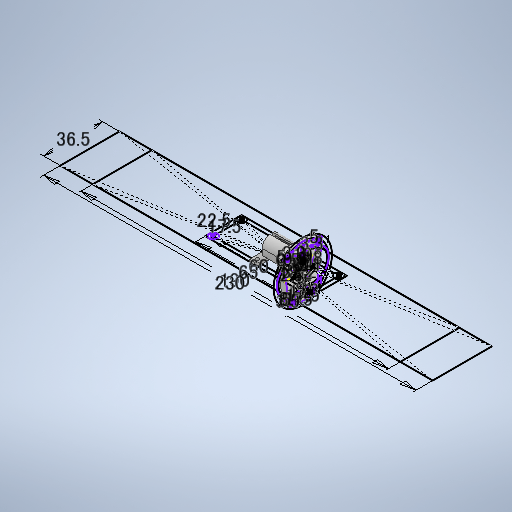
# Autodesk Inventor part: ikafly1
Saved by Autodesk Inventor 2025 (Build 290162000, 162)
## iProperties
Created: 2024-05-10
Part Number: ikafly1
Material: 一般
Document SubType Name: Modeling
Designer: Saigusa
Density: 1 g/cm^3
Appearance: 既定
Author: Saigusa
Autodesk Inventor part; units mm, degrees
ref_plane "YZ Plane" through (0, 0, 0) normal (1, 0, 0) x (0, 1, 0)
ref_plane "XZ Plane" through (0, 0, 0) normal (0, 1, 0) x (-1, 0, 0)
ref_plane "XY Plane" through (0, 0, 0) normal (0, 0, 1) x (1, 0, 0)
sketch "スケッチ2" plane through (0, 0, 0) normal (0, 1, 0) x (-1, 0, 0)
  line L0 (-32.5, -11.25) -> (32.5, -11.25)
  line L1 (32.5, -11.25) -> (32.5, 11.25)
  line L2 (32.5, 11.25) -> (-32.5, 11.25)
  line L3 (-32.5, 11.25) -> (-32.5, -11.25)
  line L4 (-32.5, -11.25) -> (32.5, 11.25) construction
  line L5 (32.5, -11.25) -> (-32.5, 11.25) construction
  line L6 (-30, -8.75) -> (30, -8.75)
  line L7 (30, -8.75) -> (30, 8.75)
  line L8 (30, 8.75) -> (-30, 8.75)
  line L9 (-30, 8.75) -> (-30, -8.75)
  line L10 (-30, -8.75) -> (30, 8.75) construction
  line L11 (30, -8.75) -> (-30, 8.75) construction
  circle A0 centre (30, 8.75) radius 2.5
  circle A1 centre (30, -8.75) radius 2.5
  circle A2 centre (-30, 8.75) radius 2.5
  circle A3 centre (-30, -8.75) radius 2.5
  line L12 (-115, -18.25) -> (115, -18.25)
  line L13 (115, -18.25) -> (115, 18.25)
  line L14 (115, 18.25) -> (-115, 18.25)
  line L15 (-115, 18.25) -> (-115, -18.25)
  line L16 (-115, -18.25) -> (115, 18.25) construction
  line L17 (115, -18.25) -> (-115, 18.25) construction
  line L18 (-95, -18.25) -> (95, -18.25)
  line L19 (95, -18.25) -> (95, 18.25)
  line L20 (95, 18.25) -> (-95, 18.25)
  line L21 (-95, 18.25) -> (-95, -18.25)
  line L22 (-95, -18.25) -> (95, 18.25) construction
  line L23 (95, -18.25) -> (-95, 18.25) construction
  point P0 (0, 0)
  dimension "d10" = 65
  dimension "d11" = 22.5
  dimension "d12" = 60
  dimension "d13" = 17.5
  dimension "d14" = 230
  dimension "d15" = 36.5
  dimension "d16" = 190
  constraints: 48 end point, 8 midpoint, 8 parallel, 4 centre point, 4 horizontal, 4 perpendicular, 4 tangent, 3 coincident, 1 point on line
  measures "d10" distance of L2.end L1.end
  measures "d11" distance of L1.end L0.end
  measures "d12" distance of L8.end L7.end
  measures "d13" distance of L7.end L6.end
  measures "d14" distance of L14.end L13.end
  measures "d15" distance of L13.end L12.end
  measures "d16" distance of L20.end L19.end
sketch "スケッチ4" plane through (0, 0, 0) normal (1, 0, 0) x (0, 1, 0)
  point P0 (0, 0)
sketch "スケッチ5" plane through (0, 0, 0) normal (1, 0, 0) x (0, 1, 0)
  circle A0 centre (0, 0) radius 18.25
  line L0 (0, 0) -> (0, 6)
  line L1 (0, 6) -> (0, -6)
  circle A1 centre (0, 6) radius 3
  circle A2 centre (0, -6) radius 9
  circle A3 centre (0, 6) radius 9
  circle A4 centre (0, -6) radius 3
  line L2 (0, 6) -> (5.2915, 0)
  circle A5 centre (5.2915, 0) radius 5
  circle A6 centre (5.2915, 0) radius 4.5
  circle A7 centre (5.2915, 0) radius 5.5
  line L3 (0, 0) -> (0, 11.25)
  line L4 (0, 11.25) -> (0, -11.25)
  line L5 (5.2915, 5.5) -> (5.2915, -5.5)
  line L6 (0, 11.25) -> (-1.2, 11.25)
  line L7 (-1.2, 11.25) -> (-1.2, -11.25)
  line L8 (-1.2, -11.25) -> (0, -11.25)
  line L9 (-1.2, 11.25) -> (-9.2, 11.25)
  line L10 (-1.2, -11.25) -> (-9.2, -11.25)
  line L11 (-9.2, -11.25) -> (-9.2, 11.25)
  line L12 (-9.2, 11.25) -> (-10.4, 11.25)
  line L13 (-10.4, 11.25) -> (-10.4, -11.25)
  line L14 (-10.4, -11.25) -> (-9.2, -11.25)
  circle A8 centre (0, 0) radius 16
  line L15 (0, 11.25) -> (1.5, 11.25)
  line L16 (1.5, 11.25) -> (1.5, -11.25)
  line L17 (1.5, -11.25) -> (0, -11.25)
  line L18 (5.2915, 5.5) -> (1.5, 5.5)
  line L19 (5.2915, -5.5) -> (1.5, -5.5)
  circle A9 centre (5.2915, 0) radius 6.6802
  point P0 (0, 1.5)
  point P1 (0, -1.5)
  point P2 (1.5, -3.9843)
  point P3 (1.5, 3.9843)
  dimension "d28" = 36.5
  dimension "d29" = 6
  dimension "d30" = 12
  dimension "d31" = 6
  dimension "d32" = 18
  dimension "d33" = 8
  dimension "d34" = 9
  dimension "d35" = 11
  dimension "d36" = 11.25
  dimension "d37" = 22.5
  dimension "d39" = 1.2
  dimension "d40" = 8
  dimension "d41" = 1.2
  dimension "d42" = 32
  dimension "d43" = 1.5
  constraints: 40 end point, 10 coincident, 9 centre point, 8 perpendicular, 7 point on line, 3 parallel, 3 point on circle, 3 tangent, 1 horizontal, 1 vertical, 3 other
  measures "d28" diameter of A0
  measures "d29" distance of L0.start L0.end
  measures "d30" distance of L0.end L1.end
  measures "d31" diameter of A1
  measures "d32" diameter of A3
  measures "d33" distance of L2.start L2.end
  measures "d34" diameter of A6
  measures "d35" diameter of A7
  measures "d36" distance of L0.start L3.end
  measures "d37" distance of L3.end L4.end
  measures "d39" distance of L3.end L6.end
  measures "d40" distance of L6.end L9.end
  measures "d41" distance of L9.end L12.end
  measures "d42" diameter of A8
  measures "d43" distance of L3.end L15.end
extrude "押し出し1" add sketch "スケッチ5" against normal blind 5 contours L0 A7 A2 A5 A3 L1 | L0 A2 A7 | A7 A3 L1 | L0 A9 L2 L16 A7 A1 | A1 A7 A2 | A7 A1 L16 A5 A2 | A4 A7 L16 A9 L1 | A3 A7 A4 | A3 A5 L16 A4 A7 | L0 L2 A9 | A7 L16 A1 | A5 L16 A2 | A2 L16 A6 A3 A5 | A9 L16 A4 L4 L1 | A4 L16 A7 | A3 L16 A5 | L3 A1 L16 A9 L2 | A9 L16 L2 | L3 L15 L16 A1 | L16 A6 | A4 L16 L17 L4 picked at (1.4091, -3.6973)
extrude "押し出し2" add sketch "スケッチ5" against normal blind 3 contours L0 A7 A2 A5 A3 L1 | A7 A1 L16 A5 A2 | A3 A5 L16 A4 A7 | A7 L16 A1 | A5 L16 A2 | A2 L16 A6 A3 A5 | A4 L16 A7 | A3 L16 A5 | L16 A7 L2 A1 | A1 A5 L16 | L16 L2 A7 | L16 A5 L2 A6 A2 | A2 A6 L16 | L16 A7 A4 L19 | L16 A5 A4 | A4 A7 L16 | L16 A6 A3 | A3 A6 L5 A5 L16 | L16 L18 A1 A7 L2 | L2 A7 A1 | A5 L5 A6 L2 | A1 A7 L5 A5 | A6 L2 A2 | A2 L2 L5 A3 A6 L16 | L16 A6 | A4 A7 L19 | A5 L5 A7 A4 | A3 L5 A6 | L18 A7 A1 | A6 L5 A2 L2 | L5 A7 A3 A5 | A5 A3 A6 L5 | A2 L5 L2 | L5 A5 A2 A7 | L5 A6 A2 A5 | L5 A2 A3 | A3 A2 A6 L5 | A6 A3 A2 L5 | A5 A2 A6 A3 | A3 A7 A2 A5 | A3 A6 A2
extrude "押し出し3" add sketch "スケッチ5" along normal blind 16.5 contours L1 A7 L0 | L0 A7 A2 A5 A3 L1 | A7 L1 A3 A9 L7 A2 L0 | L0 A2 A7 | A7 A3 L1 | A1 A9 L0 | A2 A9 A1 | L0 A9 L2 L16 A7 A1 | A1 A7 A2 | A7 A1 L16 A5 A2 | A4 A7 L16 A9 L1 | A4 A9 A3 | A3 A7 A4 | L1 A9 A4 | A3 A5 L16 A4 A7 | A7 L16 A1 | A5 L16 A2 | A2 L16 A6 A3 A5 | A4 L16 A7 | A3 L16 A5 | A9 L16 L2 | L16 A7 L2 A1 | A1 A5 L16 | L16 L2 A7 | L7 A9 | L16 A5 L2 A6 A2 | A2 A6 L16 | L16 A7 A4 L19 | L16 A5 A4 | A4 A7 L16 | L16 A6 A3 | A3 A6 L5 A5 L16 | L16 L18 A1 A7 L2 | L2 A7 A1 | A5 L5 A6 L2 | A1 A7 L5 A5 | A6 L2 A2 | A2 L2 L5 A3 A6 L16 | L16 A6 | A4 A7 L19 | A5 L5 A7 A4 | A3 L5 A6 | L18 A7 A1 | A6 L5 A2 L2 | L5 A7 A3 A5 | A5 A3 A6 L5 | A2 L5 L2 | L5 A5 A2 A7 | L5 A6 A2 A5 | L5 A2 A3 | A3 A2 A6 L5 | A6 A3 A2 L5 | A5 A2 A6 A3 | A3 A7 A2 A5 | A3 A6 A2
extrude "押し出し4" cut sketch "スケッチ5" along normal blind 16.5 contours A6 L2 A2 | A2 L2 L5 A3 A6 L16 | L16 A6 | A3 L5 A6 | A6 L5 A2 L2 | A2 L5 L2 | L5 A2 A3 | A3 A2 A6 L5 | A6 A3 A2 L5 | A3 A6 A2
extrude "押し出し5" cut sketch "スケッチ5" against normal blind 1.5 contours A6 L2 A2 | A2 L2 L5 A3 A6 L16 | L16 A6 | A3 L5 A6 | A6 L5 A2 L2 | A2 L5 L2 | L5 A2 A3 | A3 A2 A6 L5 | A6 A3 A2 L5 | A3 A6 A2
sketch "スケッチ6" plane through (16.5, 5.2915, 0) normal (1, 0, 0) x (0, 0, 1)
  line L0 (0, 5.2915) -> (6, 5.2915)
  line L1 (-11.25, 5.2915) -> (11.25, 5.2915) projected
  line L2 (6, 5.2915) -> (-6, 5.2915)
  circle A0 centre (6, 5.2915) radius 1.05
  circle A1 centre (-6, 5.2915) radius 1.05
  circle A2 centre (0, 5.2915) radius 16
  circle A3 centre (0, 0) radius 5
  line L3 (0, 0) -> (0, 3)
  line L4 (0, 3) -> (0, -5.5)
  arc A4 (-5.5, 0) -> (5.5, 0) centre (0, 0) ccw projected
  line L5 (0, 3) -> (1, 3)
  line L6 (1, 3) -> (-1, 3)
  line L7 (-1, 3) -> (-1, -5.4083)
  line L8 (1, 3) -> (1, -5.4083)
  circle A5 centre (6, 5.2915) radius 9
  circle A6 centre (-6, 5.2915) radius 9
  line L9 (0, 5.2915) -> (0, -2.7085)
  circle A7 centre (0, -2.7085) radius 8
  circle A8 centre (6, 5.2915) radius 10
  circle A9 centre (-6, 5.2915) radius 10
  line L10 (0, 5.2915) -> (0, -5.7085)
  line L11 (0, -5.7085) -> (-11.619, -5.7085)
  line L12 (0, -5.7085) -> (11.619, -5.7085)
  line L13 (0, -5.7085) -> (9.5, -5.7085)
  line L14 (9.5, -5.7085) -> (-9.5, -5.7085)
  circle A10 centre (0, 5.2915) radius 18
  line L15 (1, -5.4083) -> (1, -8.2085)
  line L16 (-1, -5.4083) -> (-1, -8.2085)
  line L17 (0, 5.2915) -> (0, 6.4915)
  line L18 (0, 6.4915) -> (0, 14.4915)
  line L19 (0, 14.4915) -> (0, 15.6915)
  line L20 (0, 15.6915) -> (-11.25, 15.6915)
  line L21 (-11.25, 15.6915) -> (11.25, 15.6915)
  line L22 (11.25, 15.6915) -> (11.25, 14.4915)
  line L23 (11.25, 14.4915) -> (0, 14.4915)
  line L24 (-11.25, 14.4915) -> (-11.25, 15.6915)
  line L25 (0, 14.4915) -> (-11.25, 14.4915)
  line L26 (0, 15.6915) -> (8.75, 15.6915)
  line L27 (8.75, 15.6915) -> (-8.75, 15.6915)
  line L28 (11.25, 15.6915) -> (11.25, 17.1915)
  line L29 (11.25, 17.1915) -> (-11.25, 17.1915)
  line L30 (-11.25, 17.1915) -> (-11.25, 15.6915)
  line L31 (6, 17.1915) -> (6, 18.6915)
  line L32 (-6, 17.1915) -> (-6, 18.6915)
  circle A11 centre (6, 18.6915) radius 2.5
  circle A12 centre (-6, 18.6915) radius 2.5
  line L33 (6, 21.1915) -> (-6, 21.1915)
  line L34 (9.5, -5.7085) -> (12, -5.7085)
  line L35 (-9.5, -5.7085) -> (-12, -5.7085)
  line L36 (6, 18.6915) -> (8.5, 18.6915)
  line L37 (-6, 18.6915) -> (-8.5, 18.6915)
  circle A13 centre (0, 0) radius 4.5
  circle A14 centre (-6, 5.2915) radius 1.5
  circle A15 centre (6, 5.2915) radius 1.5
  circle A16 centre (6, 18.6915) radius 1.65
  circle A17 centre (-6, 18.6915) radius 1.65
  line L38 (9.5, -5.7085) -> (9.5, -6.2085)
  line L39 (9.5, -6.2085) -> (-9.5, -6.2085)
  line L40 (-9.5, -6.2085) -> (-9.5, -5.7085)
  circle A18 centre (-9.5, -6.2085) radius 1.65
  circle A19 centre (9.5, -6.2085) radius 1.65
  circle A20 centre (9.5, -6.2085) radius 2.5
  circle A21 centre (-9.5, -6.2085) radius 2.5
  line L41 (-12, -6.2085) -> (-8.5, 18.6915)
  line L42 (12, -6.2085) -> (8.5, 18.6915)
  line L43 (9.5, -8.7085) -> (-9.5, -8.7085)
  line L44 (1, -8.7085) -> (1, -8.0358)
  line L45 (-1, -8.7085) -> (-1, -8.2085)
  point P0 (1, -4.3875)
  point P1 (-1, -4.3875)
  point P2 (-4.4567, 20.6583)
  point P3 (-8.495, 18.8501)
  point P4 (4.4567, 20.6583)
  point P5 (8.495, 18.8501)
  point P6 (1.7861, 21.1915)
  point P7 (-1.7861, 21.1915)
  point P8 (11.9031, -5.5193)
  point P9 (11.8759, -5.4306)
  point P10 (11.8887, -5.4164)
  dimension "d54" = 6
  dimension "d55" = 12
  dimension "d56" = 2.1
  dimension "d57" = 2.1
  dimension "d58" = 32
  dimension "d59" = 10
  dimension "d60" = 3
  dimension "d61" = 1
  dimension "d62" = 2
  dimension "d65" = 18
  dimension "d66" = 18
  dimension "d67" = 8
  dimension "d68" = 11
  dimension "d69" = 9.5
  dimension "d70" = 19
  dimension "d73" = 36
  dimension "d76" = 1.2
  dimension "d77" = 8
  dimension "d78" = 1.2
  dimension "d79" = 8.75
  dimension "d80" = 17.5
  dimension "d81" = 1.5
  dimension "d82" = 1.5
  dimension "d83" = 5
  dimension "d84" = 5
  dimension "d97" = 3
  dimension "d98" = 3
  dimension "d109" = 3.3
  dimension "d110" = 3.3
  dimension "d111" = 0.5
  dimension "d112" = 3.3
  dimension "d113" = 3.3
  dimension "d114" = 5
  dimension "d115" = 5
  constraints: 90 end point, 23 point on line, 21 centre point, 18 coincident, 13 perpendicular, 13 point on circle, 5 vertical, 3 horizontal, 2 parallel, 2 tangent
  measures "d54" distance of L0.start L0.end
  measures "d55" distance of L0.end L2.end
  measures "d56" diameter of A0
  measures "d57" diameter of A1
  measures "d58" diameter of A2
  measures "d59" diameter of A3
  measures "d60" distance of L3.start L3.end
  measures "d61" distance of L3.end L5.end
  measures "d62" distance of L5.end L6.end
  measures "d65" diameter of A5
  measures "d66" diameter of A6
  measures "d67" distance of L9.start L9.end
  measures "d68" distance of L9.start L10.end
  measures "d69" distance of L10.end L13.end
  measures "d70" distance of L13.end L14.end
  measures "d73" diameter of A10
  measures "d76" distance of L17.start L17.end
  measures "d77" distance of L17.end L18.end
  measures "d78" distance of L18.end L19.end
  measures "d79" distance of L19.end L26.end
  measures "d80" distance of L26.end L27.end
  measures "d81" distance of L21.end L28.end
  measures "d82" distance of L31.start L31.end
  measures "d83" diameter of A11
  measures "d84" diameter of A12
  measures "d97" diameter of A14
  measures "d98" diameter of A15
  measures "d109" diameter of A16
  measures "d110" diameter of A17
  measures "d111" distance of L34.start L38.end
  measures "d112" diameter of A18
  measures "d113" diameter of A19
  measures "d114" diameter of A20
  measures "d115" diameter of A21
extrude "押し出し6" cut sketch "スケッチ6" against normal blind 19.5 contours L5 L8 A6 L4 L3 | L3 L4 A5 L7 L6 | L8 A9 A5 A6 | A5 A6 A8 L7 | L8 A5 A9 | A5 A9 L4 | L4 A8 A6 | A8 A6 L7 | L8 A8 A9 A5 | A8 L8 A13 L4 | A9 L7 A6 A8 | L4 A13 L7 A9 | L7 A13 L4 A3 | A3 L4 A4 L7 | L8 A4 L4 A3 | A3 L4 A13 L8
sketch "スケッチ7" plane through (-5, 1.5, -11.25) normal (0, 1, 0) x (1, 0, 0)
  line L0 (0, 0) -> (2.5, 0)
  line L1 (5, 0) -> (0, 0) projected
  line L2 (2.5, 0) -> (2.5, -22.5)
  line L3 (5, -22.5) -> (0, -22.5) projected
  line L4 (2.5, 0) -> (2.5, -2.5)
  line L5 (2.5, -2.5) -> (2.5, -20)
  point P0 (5, -11.25)
  dimension "d87" = 2.5
  dimension "d88" = 17.5
  constraints: 8 end point, 2 midpoint, 2 point on line
  measures "d87" distance of L0.end L4.end
  measures "d88" distance of L4.end L5.end
hole "穴1" at (-2.5, 1.5, -8.75) at (-2.5, 1.5, 8.75) direction (0, -1, 0) diameter 2 end through all
fillet "フィレット1" radius 2 2 edges at (0, 0.75, -11.25) (0, 0.75, 11.25)
extrude "押し出し11" add sketch "スケッチ6" against normal blind 4 contours L17 L18 A6 L0 | A7 A5 L1 | A7 A6 A3 L9 | L0 A6 A7 | L9 A3 A5 A7 | L1 A5 L18 L17 | A6 A5 A9 L0 | L0 A9 A7 A6 | A5 A7 A8 L1 | L1 A8 A6 A5 | L9 A13 A5 A3 | A3 A6 A13 L9 | A7 A9 A3 A6 | A5 A3 A8 A7 | A9 A5 L42 L1 A15 L0 | L0 A15 L1 L42 A5 A7 A9 | L18 A9 A5 | A6 A8 L18 | A8 A7 A6 L41 L1 A14 | L1 A14 L41 A6 A8 | A3 A9 A13 A6 | A5 A13 A8 A3 | A7 A5 A3 A9 | A8 A3 A6 A7 | A15 L1 A0 L0 | L0 A0 L1 A15 | A9 A8 L23 L42 A5 | A6 L41 L25 A9 A8 | L18 L23 A8 | A9 L25 L18 | A14 L1 A1 | L1 A1 A14 | A3 A5 A13 A9 | A8 A13 A6 A3 | A7 A21 A9 L41 A6 | A6 A4 A9 A21 A7 | L23 L19 L21 L42 A8 | A8 L42 L23 | L25 L41 A9 | A9 L41 L20 L19 L25 | A6 A13 A9 A3 | A3 A9 A4 A6 | A7 A20 A8 A4 A5 | A5 L42 A8 A20 A7 | A21 A9 A7 | A7 A9 A21 | L20 L41 L29 A12 A11 L42 L21 | A5 A4 A8 A3 | A3 A8 A13 A5 | A9 A13 L7 A3 | A3 L7 A4 A9 | A20 A8 A7 | A7 A8 A20 | A9 A21 A2 L41 | A4 L16 L11 A21 A9 | A9 A21 L11 A7 | A7 L11 A18 A2 A21 A9 | A8 A4 L8 A3 | A3 L8 A13 A8 | A8 A20 L12 L15 A4 | L42 A2 A20 A8 | A8 A20 A2 L12 A19 A7 | A7 L12 A20 A8 | A2 A21 L41 | L11 A21 L39 A7 | A7 L39 A18 L11 | L11 L16 L39 A21 | A2 L35 L41 A21 | L29 A11 L42 | L41 A12 L29 | L12 A19 L39 A7 | A7 L39 A20 L12 | A20 L42 L34 A2 | A20 L39 L15 L12 | L39 A21 A7 | A7 A21 A2 A18 L39 | L39 L16 L45 L43 A7 A21 | L11 A18 A2 | A2 A18 A21 L41 L35 | A11 L29 A16 | L29 A16 L36 A11 | L36 A16 A2 A11 | A12 L37 A17 L29 | L29 A17 A12 | A12 A2 A17 L37 | L39 A19 A2 A20 A7 | A7 A20 L39 | L34 L42 A20 A2 A19 | A2 A19 L12 | A20 A7 L43 L44 L15 L39 | A7 L43 A2 A21 | A2 A16 A11 | A11 A2 A16 L29 | L29 A12 A2 L33 A11 | L29 A17 A2 A12 | A12 A2 A17 | A20 A2 L43 A7 | A2 L43 A21 | A11 A2 L33 | L33 A2 A12 | A20 L43 A2 picked at (5.1751, 14.7127) picked at (-5.1751, 14.7127)
